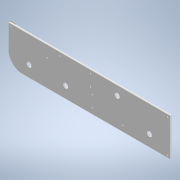
# Autodesk Inventor part: outside wall 2
Saved by Autodesk Inventor 2020 (Build 240168000, 168)
## iProperties
Created: 2020-03-07
Part Number: outside wall 2
Material: Generic
Document SubType Name: Modeling
Designer: jackm
Density: 1 g/cm^3
Appearance: Default
Author: jackm
Autodesk Inventor part; units mm, degrees
ref_plane "YZ Plane" through (0, 0, 0) normal (1, 0, 0) x (0, 1, 0)
ref_plane "XZ Plane" through (0, 0, 0) normal (0, 1, 0) x (-1, 0, 0)
ref_plane "XY Plane" through (0, 0, 0) normal (0, 0, 1) x (1, 0, 0)
ref_plane "Work Plane1" through (-137.1271, 2.9342, 0.007) normal (0, 0, 1) x (-1, 0, 0)
sketch "Sketch1" plane through (-137.1271, 2.9342, 0.007) normal (0, 0, 1) x (-1, 0, 0)
  line L0 (6.35, -6.35) -> (-444.5, -6.35) construction
  line L1 (6.35, 60.5102) -> (6.35, -6.35) construction
  arc A0 (6.35, 60.5102) -> (-31.75, 98.6102) centre (-31.75, 60.5102) ccw construction
  line L2 (-444.5, 98.6102) -> (-31.75, 98.6102) construction
  line L3 (-444.5, -6.35) -> (-444.5, 98.6102) construction
  line L4 (6.35, -6.35) -> (-444.5, -6.35)
  line L5 (-444.5, -6.35) -> (-444.5, 98.6102)
  line L6 (-444.5, 98.6102) -> (-31.75, 98.6102)
  arc A1 (6.35, 60.5102) -> (-31.75, 98.6102) centre (-31.75, 60.5102) ccw
  line L7 (6.35, -6.35) -> (6.35, 60.5102)
  circle A2 centre (0, 0) radius 1.7 construction
  circle A3 centre (-101.6148, 24.9502) radius 1.7 construction
  circle A4 centre (-222.6743, 2.9342) radius 1.9304 construction
  circle A5 centre (-222.6743, 34.9382) radius 1.9304 construction
  circle A6 centre (-227.4763, 50.9282) radius 1.9304 construction
  circle A7 centre (-227.4763, 82.9322) radius 1.9304 construction
  circle A8 centre (-313.0743, 82.9322) radius 1.9304 construction
  circle A9 centre (-137.0763, 2.9342) radius 1.9304 construction
  circle A10 centre (-438.15, 0) radius 1.7 construction
  circle A11 centre (-438.15, 92.2602) radius 1.7 construction
  circle A12 centre (-387.1214, 66.8602) radius 4.83 construction
  circle A13 centre (-51.0689, 66.8602) radius 5.2798 construction
  circle A14 centre (-153.0753, 66.9332) radius 4.15 construction
  circle A15 centre (-297.0753, 18.9332) radius 4.83 construction
  circle A16 centre (0, 0) radius 1.7
  circle A17 centre (-101.6148, 24.9502) radius 1.7
  circle A18 centre (-438.15, 0) radius 1.7
  circle A19 centre (-438.15, 92.2602) radius 1.7
  circle A20 centre (-137.0763, 2.9342) radius 1.7
  circle A21 centre (-222.6743, 2.9342) radius 1.7
  circle A22 centre (-222.6743, 34.9382) radius 1.7
  circle A23 centre (-227.4763, 50.9282) radius 1.7
  circle A24 centre (-227.4763, 82.9322) radius 1.7
  circle A25 centre (-313.0743, 82.9322) radius 1.7
  circle A26 centre (-51.0689, 66.8602) radius 6.8834
  circle A27 centre (-153.0753, 66.9332) radius 6.8834
  circle A28 centre (-297.0753, 18.9332) radius 6.8834
  circle A29 centre (-387.1214, 66.8602) radius 6.8834
  point P0 (-137.1271, 2.9342)
  dimension "d0" = 3.4
  dimension "d1" = 3.4
  dimension "d2" = 3.4
  dimension "d3" = 3.4
  dimension "d4" = 3.4
  dimension "d5" = 3.4
  dimension "d6" = 3.4
  dimension "d7" = 3.4
  dimension "d8" = 3.4
  dimension "d9" = 3.4
  dimension "d10" = 13.7668
  dimension "d11" = 13.7668
  dimension "d12" = 13.7668
  dimension "d13" = 13.7668
  constraints: 15 centre point, 15 coincident, 8 end point, 4 collinear, 2 point on circle, 1 tangent
  measures "d0" diameter of A16
  measures "d1" diameter of A17
  measures "d2" diameter of A18
  measures "d3" diameter of A19
  measures "d4" diameter of A20
  measures "d5" diameter of A21
  measures "d6" diameter of A22
  measures "d7" diameter of A23
  measures "d8" diameter of A24
  measures "d9" diameter of A25
  measures "d10" diameter of A26
  measures "d11" diameter of A27
  measures "d12" diameter of A28
  measures "d13" diameter of A29
extrude "Extrusion1" add sketch "Sketch1" along normal blind 5
body "Solid1"
